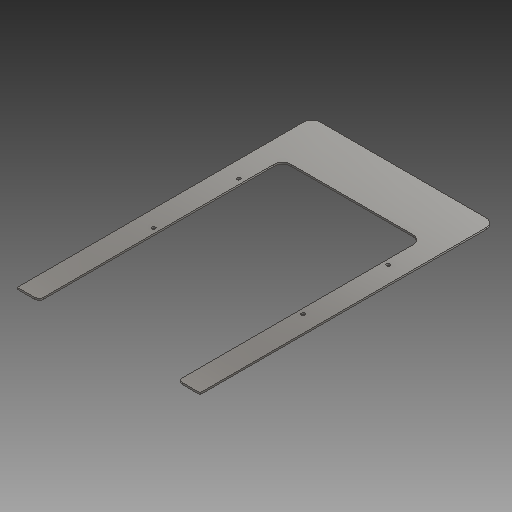
# Autodesk Inventor part: Front
Saved by Autodesk Inventor 2018 (Build 220112000, 112)
## iProperties
Created: 2017-10-08
Part Number: Front
Material: Edelstahl
Document SubType Name: Blech
Designer: jro
Density: 8 g/cm^3
Sheet Metal Rule: Standard_mm
Appearance: Halbpoliert
Mass: 63.4396 g
Surface Area: 668.249 cm^2
Volume: 63.4396 cm^3
Author: jro
Autodesk Inventor part; units mm, degrees
ref_plane "YZ Plane" through (0, 0, 0) normal (1, 0, 0) x (0, 1, 0)
ref_plane "XZ Plane" through (0, 0, 0) normal (0, 1, 0) x (-1, 0, 0)
ref_plane "XY Plane" through (0, 0, 0) normal (0, 0, 1) x (1, 0, 0)
sketch "Skizze1" plane through (0, 0, 0) normal (0, 0, 1) x (1, 0, 0)
  line L0 (106.9629, 2) -> (-106.9629, 2)
  line L1 (0, -19.6018) -> (0, 5.6106)
  line L2 (0, 2) -> (81.5, 2)
  line L3 (0, 2) -> (-81.5, 2)
  line L4 (-81.5, 2) -> (-81.5, 277)
  line L5 (81.5, 2) -> (81.5, 277)
  line L6 (71.5, 287) -> (-71.5, 287)
  arc A0 (81.5, 277) -> (71.5, 287) centre (71.5, 277) ccw
  arc A1 (-71.5, 287) -> (-81.5, 277) centre (-71.5, 277) ccw
  line L7 (-81.5, 2) -> (-106.9629, 2)
  line L8 (-106.9629, 2) -> (-106.9629, 337)
  line L9 (81.5, 2) -> (106.9629, 2)
  line L10 (106.9629, 2) -> (106.9629, 337)
  line L11 (96.9629, 347) -> (-96.9629, 347)
  arc A2 (106.9629, 337) -> (96.9629, 347) centre (96.9629, 337) ccw
  arc A3 (-96.9629, 347) -> (-106.9629, 337) centre (-96.9629, 337) ccw
  point P0 (0, 0)
  point P1 (-81.5, 287)
  point P2 (81.5, 287)
  point P3 (-106.9629, 347)
  point P4 (106.9629, 347)
  dimension "d0" = 81.5
  dimension "d1" = 81.5
  dimension "PortalHoehe" = 285
  dimension "d3" = 285
  dimension "d4" = 10
  dimension "GesammtHoehe" = 345
  dimension "d6" = 345
  dimension "d7" = 10
  measures "d0" distance of L2.start L2.end
  measures "d1" distance of L2.start L3.end
  measures "PortalHoehe" distance of L3.end point (-81.5, 287)
  measures "d3" distance of L2.end point (81.5, 287)
  measures "d4" radius of A0
  measures "GesammtHoehe" distance of L0.end point (-106.963, 347)
  measures "d6" distance of L0.start point (106.963, 347)
  measures "d7" radius of A2
extrude "Grobblech1" add sketch "Skizze1" along normal blind 2 contours L0 L5 A0 L6 A1 L4 L8 A3 L11 A2 L10
fillet "Rundung1" radius 5 2 edges at (-81.5, 2, 1) (81.5, 2, 1)
sketch "Skizze3" plane through (0, 0, 0) normal (0, 0, -1) x (-1, 0, 0)
  arc A0 (-86.5, 2) -> (-81.5, 7) centre (-86.5, 7) ccw projected
  line L0 (-81.5, 277) -> (-81.5, 7) projected
  arc A1 (-71.5, 287) -> (-81.5, 277) centre (-71.5, 277) ccw projected
  line L1 (71.5, 287) -> (-71.5, 287) projected
  arc A2 (81.5, 277) -> (71.5, 287) centre (71.5, 277) ccw projected
  line L2 (81.5, 7) -> (81.5, 277) projected
  arc A3 (81.5, 7) -> (86.5, 2) centre (86.5, 7) ccw projected
  line L3 (106.9629, 2) -> (86.5, 2) projected
  line L4 (106.9629, 337) -> (106.9629, 2) projected
  arc A4 (106.9629, 337) -> (96.9629, 347) centre (96.9629, 337) ccw projected
  line L5 (-96.9629, 347) -> (96.9629, 347) projected
  arc A5 (-96.9629, 347) -> (-106.9629, 337) centre (-96.9629, 337) ccw projected
  line L6 (-106.9629, 2) -> (-106.9629, 337) projected
  line L7 (-86.5, 2) -> (-106.9629, 2) projected
  circle A6 centre (-87.5, 142) radius 2.15
  circle A7 centre (87.5, 142) radius 2.15
  circle A8 centre (-87.5, 242) radius 2.15
  circle A9 centre (87.5, 242) radius 2.15
  point P0 (0, 0)
  dimension "Durchmesser" = 4.3
  dimension "d23" = 140
  dimension "d24" = 6
  dimension "d25" = 4.3
  dimension "d26" = 6
  dimension "d27" = 140
  dimension "d30" = 4.3
  dimension "d31" = 4.3
  dimension "d32" = 6
  dimension "d33" = 6
  dimension "d34" = 100
  dimension "d35" = 100
  constraints: 4 centre point
  measures "Durchmesser" diameter of A6
  measures "d23" distance from line of L7 A6.centre
  measures "d24" distance from line of L0 A6.centre
  measures "d25" diameter of A7
  measures "d26" distance from line of L2 A7.centre
  measures "d27" distance from line of L3 A7.centre
  measures "d30" diameter of A8
  measures "d31" diameter of A9
  measures "d32" distance from line of L0 A8.centre
  measures "d33" distance from line of L2 A9.centre
  measures "d34" distance of A7.centre A9.centre
  measures "d35" distance of A6.centre A8.centre
extrude "Extrusion3" cut sketch "Skizze3" against normal through all contours A6 | A7 | A8 | A9
equation "\"d0\" = 0.5 * PortalBreite"
equation "\"d1\" = 0.5 * PortalBreite"
equation "\"d25\" = Durchmesser"
equation "\"d26\" = d24"
equation "\"d27\" = d23"
equation "\"d30\" = Durchmesser"
equation "\"d31\" = Durchmesser"
equation "\"d32\" = d24"
equation "\"d33\" = d24"
equation "\"d35\" = d34"
equation "\"d8\" = Stärke"
equation "\"d3\" = PortalHoehe"
equation "\"d6\" = GesammtHoehe"
equation "\"PortalBreite\" = 163"
equation "\"Biegeradius\" = Stärke"
equation "\"BreiteBiegungsfreistellung\" = Stärke"
equation "\"TiefeBiegungsfreistellung\" = 0.5 * Stärke"
equation "\"GrößeEckenfreistellung\" = 4 * Stärke"
equation "\"MinimalRest\" = 2 * Stärke"
equation "\"Übergangsradius\" = Biegeradius"
equation "\"JacobiRadiusGröße\" = Biegeradius"
equation "\"Abstandsgröße\" = Stärke"
equation "\"Stärke\" = 2"
